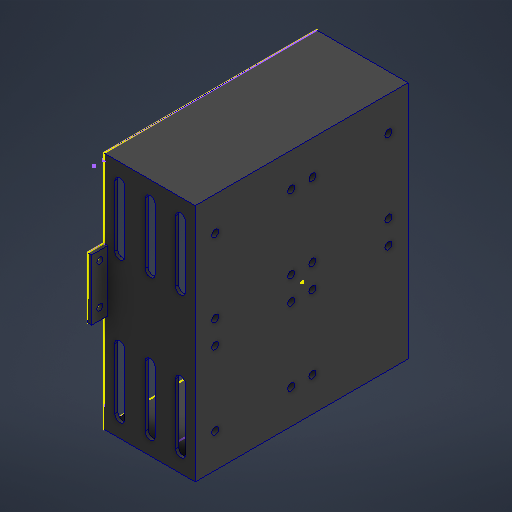
# Autodesk Inventor part: PARTE
Saved by Autodesk Inventor 2027 (Build 310192000, 192)
## iProperties
Created: 2026-06-25
Part Number: PARTE
Material: Generic
Document SubType Name: Modeling
Designer: uchiha
Density: 1 g/cm^3
Appearance: Default
Author: uchiha
Autodesk Inventor part; units mm, degrees
sketch "Sketch1" plane through (0, 0, 0) normal (1, 0, 0) x (0, 1, 0)
  circle A0 centre (-57.5, -57.5) radius 0.00002
  line L0 (59.00002, -52.5) -> (-59.00002, -52.5)
  line L1 (-59.00002, -52.5) -> (-59.00002, 52.5)
  line L2 (-59.00002, 52.5) -> (59.00002, 52.5)
  line L3 (59.00002, 52.5) -> (59.00002, -52.5)
  line L4 (57.50002, 51) -> (-57.50002, 51)
  line L5 (-57.50002, 51) -> (-57.50002, -51)
  line L6 (-57.50002, -51) -> (57.50002, -51)
  line L7 (57.50002, -51) -> (57.50002, 51)
  point P0 (0, 0)
  point P1 (55.99998, 57.5)
  point P2 (55.99998, 52.5)
  point P3 (55.99998, -52.5)
  constraints: 16 end point, 4 parallel, 2 perpendicular, 2 point on line, 1 centre point, 1 horizontal, 3 other
extrude "Extrusion1" add sketch "Sketch1" along normal blind 45
ref_plane "Work Plane1" through (25, 0, 0) normal (1, 0, 0) x (0, 1, 0)
sketch "Sketch3" plane through (25, 0, 0) normal (1, 0, 0) x (0, 1, 0)
  point P0 (0, 0)
sketch "Sketch4" plane through (25, 0, 0) normal (1, 0, 0) x (0, 1, 0)
  line L0 (-57.50002, -51) -> (-57.50002, 51)
  point P0 (0, 0)
  constraints: 2 end point
ref_plane "Work Plane3" through (0, 0, 30) normal (0, 0, 1) x (1, 0, 0)
ref_plane "Work Plane13" through (27, 0, 0) normal (1, 0, 0) x (0, 0, -1)
sketch "Sketch6" plane through (27, 0, 0) normal (1, 0, 0) x (0, 0, -1)
  point P0 (0, 0)
sketch "Sketch7" plane through (45, 0, 0) normal (1, 0, 0) x (0, 0, -1)
  point P0 (0, 0)
ref_plane "Work Plane15" through (27, 0, 0) normal (1, 0, 0) x (0, 0, -1)
sketch "Sketch9" plane through (27, 0, 0) normal (1, 0, 0) x (0, 0, -1)
  line L0 (-51, 57.50002) -> (51, 57.50002)
  line L1 (51, 39.692184) -> (51, 55.423577)
  line L2 (51, 57.50002) -> (51, -57.50002)
  point P0 (51, -57.50002)
  constraints: 2 end point, 1 vertical, 1 other
ref_plane "Work Plane14" through (27, 0, 0) normal (1, 0, 0) x (0, 0, -1)
sketch "Sketch11" plane through (27, 0, 0) normal (1, 0, 0) x (0, 0, -1)
  line L0 (-394.421672, 97.846313) -> (-394.421672, 140.846313)
  line L1 (-394.421672, 140.846313) -> (-351.421672, 140.846313)
  line L2 (-394.421672, 97.846313) -> (-351.421672, 97.846313)
  line L3 (-351.421672, 97.846313) -> (-351.421672, 140.846313)
  line L4 (-351.421672, 140.846313) -> (-394.421672, 140.846313)
  line L5 (-394.421672, 140.846313) -> (-394.421672, 97.846313)
  circle A0 centre (-391.664859, 101.160601) radius 1.75
  circle A1 centre (-391.664859, 101.160601) radius 1.75
  circle A2 centre (-391.664859, 101.160601) radius 2.545638
  line L6 (-372.921672, 140.846313) -> (-372.921672, 97.846313)
  line L7 (-394.421672, 119.346313) -> (-351.421672, 119.346313)
  circle A3 centre (-391.664859, 137.532025) radius 1.75
  circle A4 centre (-391.664859, 137.532025) radius 2.545638
  circle A5 centre (-354.178484, 101.160601) radius 2.545638
  circle A6 centre (-354.178484, 101.160601) radius 1.75
  circle A7 centre (-354.178484, 137.532025) radius 2.545638
  circle A8 centre (-354.178484, 137.532025) radius 1.75
  circle A9 centre (-343.664859, 101.160601) radius 1.75
  circle A10 centre (-343.664859, 101.160601) radius 2.545638
  line L8 (-346.421672, 97.846313) -> (-346.421672, 140.846313)
  circle A11 centre (-343.664859, 137.532025) radius 1.75
  circle A12 centre (-343.664859, 137.532025) radius 2.545638
  line L9 (-324.921672, 140.846313) -> (-324.921672, 97.846313)
  circle A13 centre (-306.178484, 101.160601) radius 1.75
  circle A14 centre (-306.178484, 101.160601) radius 1.75
  line L10 (-303.421672, 97.846313) -> (-346.421672, 97.846313)
  circle A15 centre (-306.178484, 101.160601) radius 2.545638
  line L11 (-303.421672, 119.346313) -> (-346.421672, 119.346313)
  line L12 (-303.421672, 140.846313) -> (-346.421672, 140.846313)
  line L13 (-346.421672, 140.846313) -> (-303.421672, 140.846313)
  circle A16 centre (-306.178484, 137.532025) radius 1.75
  circle A17 centre (-306.178484, 137.532025) radius 2.545638
  line L14 (-303.421672, 97.846313) -> (-303.421672, 140.846313)
  line L15 (-303.421672, 140.846313) -> (-303.421672, 97.846313)
  line L16 (-294.883416, 95.346313) -> (-402.959928, 95.346313)
  circle A18 centre (-354.178484, 89.532025) radius 1.75
  circle A19 centre (-354.178484, 89.532025) radius 2.545638
  line L17 (-351.421672, 92.846313) -> (-351.421672, 49.846313)
  circle A20 centre (-354.178484, 53.160601) radius 1.75
  circle A21 centre (-354.178484, 53.160601) radius 2.545638
  line L18 (-372.921672, 49.846313) -> (-372.921672, 92.846313)
  circle A22 centre (-391.664859, 89.532025) radius 1.75
  circle A23 centre (-391.664859, 89.532025) radius 1.75
  line L19 (-394.421672, 92.846313) -> (-351.421672, 92.846313)
  circle A24 centre (-391.664859, 89.532025) radius 2.545638
  line L20 (-394.421672, 71.346313) -> (-351.421672, 71.346313)
  line L21 (-394.421672, 49.846313) -> (-351.421672, 49.846313)
  line L22 (-351.421672, 49.846313) -> (-394.421672, 49.846313)
  circle A25 centre (-391.664859, 53.160601) radius 1.75
  circle A26 centre (-391.664859, 53.160601) radius 2.545638
  line L23 (-394.421672, 92.846313) -> (-394.421672, 49.846313)
  line L24 (-394.421672, 49.846313) -> (-394.421672, 92.846313)
  circle A27 centre (-343.664859, 89.532025) radius 1.75
  circle A28 centre (-343.664859, 53.160601) radius 1.75
  circle A29 centre (-343.664859, 89.532025) radius 2.545638
  circle A30 centre (-343.664859, 53.160601) radius 2.545638
  line L25 (-324.921672, 49.846313) -> (-324.921672, 92.846313)
  circle A31 centre (-306.178484, 89.532025) radius 1.75
  circle A32 centre (-306.178484, 89.532025) radius 1.75
  line L26 (-303.421672, 92.846313) -> (-346.421672, 92.846313)
  line L27 (-303.421672, 92.846313) -> (-303.421672, 49.846313)
  line L28 (-303.421672, 49.846313) -> (-303.421672, 92.846313)
  circle A33 centre (-306.178484, 89.532025) radius 2.545638
  line L29 (-303.421672, 71.346313) -> (-346.421672, 71.346313)
  circle A34 centre (-306.178484, 53.160601) radius 1.75
  circle A35 centre (-306.178484, 53.160601) radius 2.545638
  line L30 (-303.421672, 49.846313) -> (-346.421672, 49.846313)
  line L31 (-346.421672, 49.846313) -> (-303.421672, 49.846313)
  line L32 (-346.421672, 92.846313) -> (-346.421672, 49.846313)
  line L33 (-293.921672, 40.346313) -> (-403.921672, 150.346313) construction
  circle A36 centre (-4.06596, 6.500376) radius 1.75
  circle A37 centre (-4.06596, 6.500376) radius 2.545638
  line L34 (-1.309148, 3.186088) -> (-1.309148, 46.186088)
  circle A38 centre (-4.06596, 42.8718) radius 1.75
  circle A39 centre (-4.06596, 42.8718) radius 2.545638
  line L35 (-22.809148, 46.186088) -> (-22.809148, 3.186088)
  circle A40 centre (-41.552335, 6.500376) radius 1.75
  circle A41 centre (-41.552335, 6.500376) radius 1.75
  line L36 (-44.309148, 3.186088) -> (-1.309148, 3.186088)
  circle A42 centre (-41.552335, 6.500376) radius 2.545638
  line L37 (-44.309148, 24.686088) -> (-1.309148, 24.686088)
  line L38 (-44.309148, 46.186088) -> (-1.309148, 46.186088)
  line L39 (-1.309148, 46.186088) -> (-44.309148, 46.186088)
  circle A43 centre (-41.552335, 42.8718) radius 1.75
  circle A44 centre (-41.552335, 42.8718) radius 2.545638
  line L40 (-44.309148, 3.186088) -> (-44.309148, 46.186088)
  line L41 (-44.309148, 46.186088) -> (-44.309148, 3.186088)
  circle A45 centre (6.447665, 6.500376) radius 1.75
  circle A46 centre (6.447665, 42.8718) radius 1.75
  circle A47 centre (6.447665, 6.500376) radius 2.545638
  circle A48 centre (6.447665, 42.8718) radius 2.545638
  line L42 (25.190852, 46.186088) -> (25.190852, 3.186088)
  circle A49 centre (43.93404, 6.500376) radius 1.75
  circle A50 centre (43.93404, 6.500376) radius 1.75
  line L43 (46.690852, 3.186088) -> (3.690852, 3.186088)
  line L44 (46.690852, 3.186088) -> (46.690852, 46.186088)
  line L45 (46.690852, 46.186088) -> (46.690852, 3.186088)
  circle A51 centre (43.93404, 6.500376) radius 2.545638
  line L46 (46.690852, 24.686088) -> (3.690852, 24.686088)
  circle A52 centre (43.93404, 42.8718) radius 1.75
  circle A53 centre (43.93404, 42.8718) radius 2.545638
  line L47 (46.690852, 46.186088) -> (3.690852, 46.186088)
  line L48 (3.690852, 46.186088) -> (46.690852, 46.186088)
  line L49 (3.690852, 3.186088) -> (3.690852, 46.186088)
  line L50 (55.229108, 0.686088) -> (-52.847404, 0.686088)
  circle A54 centre (43.93404, -5.1282) radius 1.75
  circle A55 centre (43.93404, -5.1282) radius 1.75
  circle A56 centre (43.93404, -5.1282) radius 2.545638
  line L51 (-44.309148, -23.313912) -> (-1.309148, -23.313912)
  line L52 (-44.309148, -1.813912) -> (-44.309148, -44.813912)
  line L53 (-44.309148, -44.813912) -> (-44.309148, -1.813912)
  line L54 (-22.809148, -44.813912) -> (-22.809148, -1.813912)
  line L55 (-1.309148, -1.813912) -> (-1.309148, -44.813912)
  circle A57 centre (-4.06596, -41.499624) radius 1.75
  circle A58 centre (-4.06596, -41.499624) radius 2.545638
  line L56 (-44.309148, -44.813912) -> (-1.309148, -44.813912)
  line L57 (-1.309148, -44.813912) -> (-44.309148, -44.813912)
  circle A59 centre (-41.552335, -41.499624) radius 1.75
  circle A60 centre (-41.552335, -41.499624) radius 2.545638
  circle A61 centre (6.447665, -5.1282) radius 1.75
  circle A62 centre (6.447665, -5.1282) radius 2.545638
  line L58 (46.690852, -1.813912) -> (3.690852, -1.813912)
  circle A63 centre (43.93404, -41.499624) radius 1.75
  circle A64 centre (43.93404, -41.499624) radius 2.545638
  line L59 (46.690852, -1.813912) -> (46.690852, -44.813912)
  line L60 (46.690852, -44.813912) -> (46.690852, -1.813912)
  line L61 (46.690852, -23.313912) -> (3.690852, -23.313912)
  line L62 (25.190852, -44.813912) -> (25.190852, -1.813912)
  line L63 (46.690852, -44.813912) -> (3.690852, -44.813912)
  line L64 (3.690852, -44.813912) -> (46.690852, -44.813912)
  circle A65 centre (6.447665, -41.499624) radius 1.75
  circle A66 centre (6.447665, -41.499624) radius 2.545638
  line L65 (3.690852, -1.813912) -> (3.690852, -44.813912)
  circle A67 centre (-41.552335, -5.1282) radius 1.75
  circle A68 centre (-41.552335, -5.1282) radius 1.75
  circle A69 centre (-41.552335, -5.1282) radius 2.545638
  circle A70 centre (-4.06596, -5.1282) radius 1.75
  circle A71 centre (-4.06596, -5.1282) radius 2.545638
  line L66 (-44.309148, -1.813912) -> (-1.309148, -1.813912)
  point P0 (-348.921672, 95.346313)
  point P1 (1.190852, 0.686088)
  dimension "d71" = 5
  dimension "d80" = 5
  constraints: 134 end point, 72 centre point, 68 symmetric about line, 16 coincident, 11 midpoint, 6 perpendicular, 4 horizontal, 4 parallel, 48 other
  measures "d71" distance between parallel lines of L10 L26
  measures "d80" distance between parallel lines of L43 L58
sketch "Sketch13" plane through (0, 0, 0) normal (-1, 0, 0) x (0, 0, 1)
  line L0 (-52.5, -59.00002) -> (-52.5, 59.00002)
  line L1 (-52.5, -9.537508) -> (-60.5, -9.537508)
  line L2 (-60.5, -9.537508) -> (-60.5, 20.462492)
  line L3 (-60.5, 20.462492) -> (-52.5, 20.462492)
  line L4 (-52.5, 20.462492) -> (-52.5, -9.537508)
  line L5 (0, 33.472207) -> (0, -33.472207)
  line L6 (52.5, -9.537508) -> (60.5, -9.537508)
  line L7 (60.5, -9.537508) -> (60.5, 20.462492)
  line L8 (60.5, 20.462492) -> (52.5, 20.462492)
  line L9 (52.5, 20.462492) -> (52.5, -9.537508)
  line L10 (-52.5, 20.462492) -> (-52.5, -9.537508)
  point P0 (0, 0)
  dimension "d87" = 8
  dimension "d88" = 30
  constraints: 20 end point, 4 symmetric about line, 2 parallel, 2 perpendicular, 1 collinear, 1 horizontal, 1 midpoint, 1 point on line, 1 vertical
  measures "d87" distance of L2.end L3.end
  measures "d88" distance of L1.end L2.end
extrude "Extrusion12" add sketch "Sketch13" against normal blind 2
sketch "Sketch15" plane through (0, 0, 0) normal (-1, 0, 0) x (0, 0, 1)
  line L0 (52.5, 20.462492) -> (60.5, 20.462492)
  line L1 (56.5, 20.462492) -> (56.5, -9.537508)
  line L2 (60.5, -9.537508) -> (52.5, -9.537508)
  line L3 (60.5, 20.462492) -> (60.5, -9.537508)
  line L4 (52.5, 59.00002) -> (52.5, -59.00002)
  line L5 (-52.5, 20.462492) -> (-60.5, 20.462492)
  line L6 (-56.5, 20.462492) -> (-56.5, -9.537508)
  line L7 (-52.5, -9.537508) -> (-60.5, -9.537508)
  line L8 (-60.5, 20.462492) -> (-60.5, -9.537508)
  line L9 (-52.5, -59.00002) -> (-52.5, 59.00002)
  circle A0 centre (-56.5, -3.90727) radius 1.5
  circle A1 centre (-56.5, 16.09273) radius 1.5
  line L10 (0, 0) -> (0, -36.285486)
  circle A2 centre (56.5, -3.90727) radius 1.5
  circle A3 centre (56.5, 16.09273) radius 1.5
  dimension "d92" = 3
  dimension "d93" = 3
  dimension "d94" = 20
  constraints: 6 end point, 4 centre point, 4 midpoint, 2 point on line, 2 symmetric about line, 1 vertical, 2 other
  measures "d92" diameter of A0
  measures "d93" diameter of A1
  measures "d94" distance of A1.centre A0.centre
extrude "Extrusion13" cut sketch "Sketch15" along normal mid plane 45 contours A3 L1 | L1 A3 | A2 L1 | L1 A2 | A1 L6 | L6 A1 | A0 L6 | L6 A0
ref_plane "Work Plane16" through (45, 0, -51) normal (0.7071068, 0, -0.7071068) x (0, 1, 0)
sketch "Sketch16" plane through (45, 0, 0) normal (1, 0, 0) x (0, 0, -1)
  line L0 (51, 57.50002) -> (51, -57.50002)
  line L1 (-51, -57.50002) -> (51, -57.50002)
  line L2 (51, -57.50002) -> (51, 57.50002)
  line L3 (51, 57.50002) -> (-51, 57.50002)
  line L4 (-51, 57.50002) -> (-51, -57.50002)
  line L5 (-51, -57.50002) -> (51, 57.50002) construction
  line L6 (51, -57.50002) -> (-51, 57.50002) construction
  point P0 (0, 0)
  point P1 (51, -57.50002)
  constraints: 12 end point, 2 midpoint, 2 parallel, 1 horizontal, 1 perpendicular
extrude "Extrusion14" add sketch "Sketch16" against normal blind 2.5
sketch "Sketch17" plane through (45, 0, 0) normal (1, 0, 0) x (0, 0, -1)
  point P0 (0, 0)
sketch "Sketch18" plane through (45, 0, 0) normal (1, 0, 0) x (0, 0, -1)
  circle A0 centre (-42.662382, 42.266518) radius 1.75
  circle A1 centre (-42.662382, 42.266518) radius 2.545638
  circle A2 centre (-42.662382, 5.895094) radius 1.75
  circle A3 centre (-42.662382, 5.895094) radius 1.75
  circle A4 centre (-42.662382, 5.895094) radius 2.545638
  line L0 (-45.419194, 2.580806) -> (-45.419194, 45.580806)
  line L1 (-45.419194, 45.580806) -> (-45.419194, 2.580806)
  circle A5 centre (-5.176007, 5.895094) radius 1.75
  line L2 (-23.919194, 45.580806) -> (-23.919194, 2.580806)
  line L3 (-45.419194, 45.580806) -> (-2.419194, 45.580806)
  line L4 (-2.419194, 45.580806) -> (-45.419194, 45.580806)
  line L5 (-45.419194, 2.580806) -> (-2.419194, 2.580806)
  line L6 (-45.419194, 24.080806) -> (-2.419194, 24.080806)
  circle A6 centre (-5.176007, 5.895094) radius 2.545638
  line L7 (-2.419194, 2.580806) -> (-2.419194, 45.580806)
  circle A7 centre (5.337618, -5.733482) radius 2.545638
  circle A8 centre (-5.176007, 42.266518) radius 1.75
  circle A9 centre (-5.176007, 42.266518) radius 2.545638
  circle A10 centre (5.337618, 5.895094) radius 1.75
  circle A11 centre (5.337618, 42.266518) radius 1.75
  circle A12 centre (5.337618, 5.895094) radius 2.545638
  line L8 (2.580806, 2.580806) -> (2.580806, 45.580806)
  circle A13 centre (5.337618, 42.266518) radius 2.545638
  line L9 (24.080806, 45.580806) -> (24.080806, 2.580806)
  circle A14 centre (42.823993, 5.895094) radius 1.75
  circle A15 centre (42.823993, 5.895094) radius 1.75
  circle A16 centre (42.823993, 5.895094) radius 2.545638
  line L10 (45.580806, 2.580806) -> (2.580806, 2.580806)
  line L11 (45.580806, 2.580806) -> (45.580806, 45.580806)
  line L12 (45.580806, 45.580806) -> (45.580806, 2.580806)
  line L13 (45.580806, 45.580806) -> (2.580806, 45.580806)
  line L14 (2.580806, 45.580806) -> (45.580806, 45.580806)
  line L15 (45.580806, 24.080806) -> (2.580806, 24.080806)
  circle A17 centre (42.823993, 42.266518) radius 1.75
  circle A18 centre (42.823993, 42.266518) radius 2.545638
  circle A19 centre (5.337618, -42.104906) radius 2.545638
  line L16 (2.580806, -2.419194) -> (2.580806, -45.419194)
  circle A20 centre (42.823993, -5.733482) radius 1.75
  circle A21 centre (42.823993, -5.733482) radius 1.75
  circle A22 centre (42.823993, -5.733482) radius 2.545638
  line L17 (45.580806, -2.419194) -> (2.580806, -2.419194)
  line L18 (24.080806, -45.419194) -> (24.080806, -2.419194)
  line L19 (45.580806, -23.919194) -> (2.580806, -23.919194)
  line L20 (45.580806, -45.419194) -> (2.580806, -45.419194)
  line L21 (2.580806, -45.419194) -> (45.580806, -45.419194)
  line L22 (45.580806, -2.419194) -> (45.580806, -45.419194)
  line L23 (45.580806, -45.419194) -> (45.580806, -2.419194)
  circle A23 centre (42.823993, -42.104906) radius 1.75
  circle A24 centre (42.823993, -42.104906) radius 2.545638
  line L24 (-2.419194, -2.419194) -> (-2.419194, -45.419194)
  line L25 (-23.919194, -45.419194) -> (-23.919194, -2.419194)
  line L26 (-45.419194, -23.919194) -> (-2.419194, -23.919194)
  line L27 (-45.419194, -2.419194) -> (-45.419194, -45.419194)
  line L28 (-45.419194, -45.419194) -> (-45.419194, -2.419194)
  circle A25 centre (-5.176007, -42.104906) radius 1.75
  circle A26 centre (-42.662382, -42.104906) radius 1.75
  circle A27 centre (5.337618, -5.733482) radius 1.75
  circle A28 centre (-5.176007, -5.733482) radius 1.75
  circle A29 centre (-5.176007, -5.733482) radius 2.545638
  circle A30 centre (-42.662382, -5.733482) radius 1.75
  circle A31 centre (-42.662382, -5.733482) radius 1.75
  line L29 (-45.419194, -2.419194) -> (-2.419194, -2.419194)
  circle A32 centre (-42.662382, -5.733482) radius 2.545638
  circle A33 centre (5.337618, -42.104906) radius 1.75
  circle A34 centre (-5.176007, -42.104906) radius 2.545638
  line L30 (-45.419194, -45.419194) -> (-2.419194, -45.419194)
  line L31 (-2.419194, -45.419194) -> (-45.419194, -45.419194)
  circle A35 centre (-42.662382, -42.104906) radius 2.545638
  point P0 (0, 0)
  point P1 (0.080806, 0.080806)
  dimension "d101" = 5
  constraints: 64 end point, 36 centre point, 8 coincident, 4 midpoint, 4 symmetric about line, 3 perpendicular, 2 parallel, 1 horizontal, 6 other
  measures "d101" distance between parallel lines of L10 L17
extrude "Extrusion15" cut sketch "Sketch18" against normal blind 2.5 contours A0 | A2 | A5 | A8 | A10 | A11 | A14 | A17 | A20 | A25 | A26 | A27 | A28 | A30 | A33
sketch "Sketch20" plane through (0, 0, 0) normal (-1, 0, 0) x (0, 0, 1)
  circle A0 centre (56.5, -3.90727) radius 1.5
  circle A1 centre (-56.5, 16.09273) radius 1.5
  circle A2 centre (56.5, 16.09273) radius 1.5
  circle A3 centre (-56.5, -3.90727) radius 1.5
  line L0 (52.5, 59.00002) -> (52.5, 20.462492)
  line L1 (-52.5, 59.00002) -> (52.5, 59.00002)
  line L2 (-52.5, 20.462492) -> (-52.5, 59.00002)
  line L3 (-52.5, 20.462492) -> (-60.5, 20.462492)
  line L4 (-60.5, 20.462492) -> (-60.5, -9.537508)
  line L5 (-60.5, -9.537508) -> (-52.5, -9.537508)
  line L6 (-52.5, -59.00002) -> (-52.5, -9.537508)
  line L7 (52.5, -59.00002) -> (-52.5, -59.00002)
  line L8 (52.5, -9.537508) -> (52.5, -59.00002)
  line L9 (52.5, -9.537508) -> (60.5, -9.537508)
  line L10 (60.5, -9.537508) -> (60.5, 20.462492)
  line L11 (60.5, 20.462492) -> (52.5, 20.462492)
  line L12 (51, -57.50002) -> (51, 57.50002)
  line L13 (-51, -57.50002) -> (51, -57.50002)
  line L14 (-51, 57.50002) -> (-51, -57.50002)
  line L15 (51, 57.50002) -> (-51, 57.50002)
  line L16 (-60.559407, 20.521899) -> (-52.559407, 20.521899)
  line L17 (-52.559407, 20.521899) -> (-52.559407, 59.059427)
  line L18 (-52.559407, 59.059427) -> (52.559407, 59.059427)
  line L19 (52.559407, 59.059427) -> (52.559407, 20.521899)
  line L20 (52.559407, 20.521899) -> (60.559407, 20.521899)
  line L21 (52.559407, -9.596915) -> (52.559407, -59.059427)
  line L22 (52.559407, -59.059427) -> (-52.559407, -59.059427)
  line L23 (-52.559407, -59.059427) -> (-52.559407, -9.596915)
  line L24 (-52.559407, -9.596915) -> (-60.559407, -9.596915)
  point P0 (0, 0)
  constraints: 18 end point, 7 other
sketch "Sketch23" plane through (0, -59.00002, 52.5) normal (0, 0, 1) x (1, 0, 0)
  line L0 (45, 0) -> (45, 118.000041)
  line L1 (45, 59.00002) -> (0, 59.00002)
  line L2 (7.798622, 9.240611) -> (7.798622, 39.240611) construction
  line L3 (10.298622, 9.240611) -> (10.298622, 39.240611)
  line L4 (5.298622, 39.240611) -> (5.298622, 9.240611)
  arc A0 (5.298622, 9.240611) -> (10.298622, 9.240611) centre (7.798622, 9.240611) ccw
  arc A1 (10.298622, 39.240611) -> (5.298622, 39.240611) centre (7.798622, 39.240611) ccw
  line L5 (22.798622, 9.240611) -> (22.798622, 39.240611) construction
  line L6 (25.298622, 9.240611) -> (25.298622, 39.240611)
  line L7 (20.298622, 39.240611) -> (20.298622, 9.240611)
  arc A2 (20.298622, 9.240611) -> (25.298622, 9.240611) centre (22.798622, 9.240611) ccw
  arc A3 (25.298622, 39.240611) -> (20.298622, 39.240611) centre (22.798622, 39.240611) ccw
  line L8 (37.798622, 9.240611) -> (37.798622, 39.240611) construction
  line L9 (40.298622, 9.240611) -> (40.298622, 39.240611)
  line L10 (35.298622, 39.240611) -> (35.298622, 9.240611)
  arc A4 (35.298622, 9.240611) -> (40.298622, 9.240611) centre (37.798622, 9.240611) ccw
  arc A5 (40.298622, 39.240611) -> (35.298622, 39.240611) centre (37.798622, 39.240611) ccw
  line L11 (7.798622, 108.759429) -> (7.798622, 78.759429) construction
  line L12 (10.298622, 108.759429) -> (10.298622, 78.759429)
  line L13 (5.298622, 78.759429) -> (5.298622, 108.759429)
  arc A6 (10.298622, 108.759429) -> (5.298622, 108.759429) centre (7.798622, 108.759429) ccw
  arc A7 (5.298622, 78.759429) -> (10.298622, 78.759429) centre (7.798622, 78.759429) ccw
  line L14 (22.798622, 108.759429) -> (22.798622, 78.759429) construction
  line L15 (25.298622, 108.759429) -> (25.298622, 78.759429)
  line L16 (20.298622, 78.759429) -> (20.298622, 108.759429)
  arc A8 (25.298622, 108.759429) -> (20.298622, 108.759429) centre (22.798622, 108.759429) ccw
  arc A9 (20.298622, 78.759429) -> (25.298622, 78.759429) centre (22.798622, 78.759429) ccw
  line L17 (37.798622, 108.759429) -> (37.798622, 78.759429) construction
  line L18 (40.298622, 108.759429) -> (40.298622, 78.759429)
  line L19 (35.298622, 78.759429) -> (35.298622, 108.759429)
  arc A10 (40.298622, 108.759429) -> (35.298622, 108.759429) centre (37.798622, 108.759429) ccw
  arc A11 (35.298622, 78.759429) -> (40.298622, 78.759429) centre (37.798622, 78.759429) ccw
  point P0 (7.798622, 24.240611)
  point P1 (22.798622, 24.240611)
  point P2 (37.798622, 24.240611)
  point P3 (7.798622, 93.759429)
  point P4 (22.798622, 93.759429)
  point P5 (37.798622, 93.759429)
  dimension "d106" = 30
  dimension "d107" = 5
  dimension "d110" = 15
  constraints: 50 end point, 24 point on circle, 21 symmetric about line, 12 centre point, 4 tangent, 2 horizontal, 2 midpoint, 1 parallel, 1 vertical, 30 other
  measures "d106" distance of L2.start L2.end
  measures "d107" diameter of A1
  measures "d110" distance of L3.start L6.start
extrude "Extrusion16" cut sketch "Sketch23" against normal blind 200
body "Solid1"
